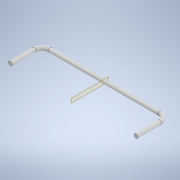
# Autodesk Inventor part: stabbar_u5
Saved by Autodesk Inventor 2022 (Build 260153000, 153)
## iProperties
Created: 2022-02-12
Part Number: stabbar_u5
Material: Generic
Document SubType Name: Modeling
Designer: Yazawa
Density: 1 g/cm^3
Appearance: Default
Author: Yazawa
Autodesk Inventor part; units mm, degrees
ref_plane "XZ Plane" through (0, 0, 0) normal (0, 1, 0) x (-1, 0, 0)
ref_plane "XY Plane" through (0, 0, 0) normal (0, 0, 1) x (1, 0, 0)
sketch "スケッチ1" plane through (0, 0, 0) normal (0, 0, 1) x (1, 0, 0)
  circle A0 centre (-25.4, 0) radius 0.8
  point P0 (0, 0)
  dimension "d0" = 1.6
  dimension "d3" = 25.4
  constraints: 1 centre point, 1 horizontal alignment
  measures "d0" diameter of A0
  measures "d3" distance of point (0, 0) A0.centre
sketch "スケッチ2" plane through (0, 0, 0) normal (0, 1, 0) x (-1, 0, 0)
  line L0 (25.4, 0) -> (25.4, -9.625)
  line L1 (22.225, -12.8) -> (-22.225, -12.8)
  line L2 (-25.4, -9.625) -> (-25.4, 0)
  arc A0 (22.225, -12.8) -> (25.4, -9.625) centre (22.225, -9.625) ccw
  arc A1 (-25.4, -9.625) -> (-22.225, -12.8) centre (-22.225, -9.625) ccw
  point P0 (0, 0)
  point P1 (0, -12.8)
  dimension "d1" = 3.175
  dimension "d2" = 12.8
  constraints: 6 end point, 4 point on circle, 4 tangent, 2 centre point, 2 perpendicular, 1 equal radius, 1 horizontal alignment, 1 midpoint, 1 vertical, 1 vertical alignment
  measures "d1" radius of A0
  measures "d2" distance from line of L0.start L1
sweep "スイープ1" add profiles "スケッチ1" path "スケッチ2"
